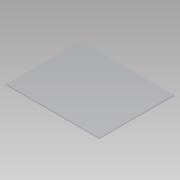
# Autodesk Inventor part: optix 8x10 window
Saved by Autodesk Inventor 2015 (Build 190159000, 159)
## iProperties
Created: 2015-05-21
Part Number: optix 8x10 window
Material: Polycarbonate, Clear
Document SubType Name: Modeling
Designer: Joe Sheldon
Density: 1.2 g/cm^3
Appearance: Polycarbonate - Clear
Author: Joe Sheldon
Autodesk Inventor part; units mm, degrees
ref_plane "YZ Plane" through (0, 0, 0) normal (1, 0, 0) x (0, 1, 0)
ref_plane "XZ Plane" through (0, 0, 0) normal (0, 1, 0) x (-1, 0, 0)
ref_plane "XY Plane" through (0, 0, 0) normal (0, 0, 1) x (1, 0, 0)
sketch "Sketch1" plane through (0, 0, 0) normal (0, 1, 0) x (-1, 0, 0)
  line L0 (-127, 101.6) -> (-127, -101.6)
  line L1 (-127, -101.6) -> (127, -101.6)
  line L2 (127, -101.6) -> (127, 101.6)
  line L3 (127, 101.6) -> (-127, 101.6)
  line L4 (-127, 101.6) -> (127, -101.6) construction
  line L5 (-127, -101.6) -> (127, 101.6) construction
  line L6 (-127, 101.6) -> (76.2, 101.6) construction
  point P0 (0, 0)
  dimension "d0" = 203.2
  dimension "d1" = 90
  dimension "d2" = 254
  constraints: 14 end point, 2 midpoint, 2 parallel, 2 perpendicular, 1 horizontal, 1 vertical
  measures "d0" distance of L0.start L0.end
  measures "d1" angle of L0 L6
  measures "d2" distance of L1.end L0.end
extrude "Extrusion1" add sketch "Sketch1" along normal blind 2.032
body "Solid1"
